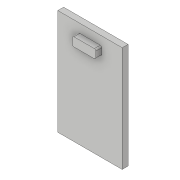
# Autodesk Inventor part: door
Saved by Autodesk Inventor 2017 (Build 210142000, 142)
## iProperties
Created: 2018-11-30
Part Number: door
Material: Generic
Document SubType Name: Modeling
Designer: jpb34
Density: 1 g/cm^3
Appearance: Default
Author: jpb34
Autodesk Inventor part; units mm, degrees
ref_plane "YZ Plane" through (0, 0, 0) normal (1, 0, 0) x (0, 1, 0)
ref_plane "XZ Plane" through (0, 0, 0) normal (0, 1, 0) x (-1, 0, 0)
ref_plane "XY Plane" through (0, 0, 0) normal (0, 0, 1) x (1, 0, 0)
sketch "Sketch1" plane through (0, 0, 0) normal (0, 0, 1) x (1, 0, 0)
  line L0 (-69.85, 114.3) -> (69.85, 114.3)
  line L1 (69.85, 114.3) -> (69.85, -114.3)
  line L2 (69.85, -114.3) -> (-69.85, -114.3)
  line L3 (-69.85, -114.3) -> (-69.85, 114.3)
  point P0 (0, 0)
  dimension "d0" = 139.7
  dimension "d1" = 228.6
  dimension "d2" = 114.3
  dimension "d3" = 69.85
  constraints: 8 end point, 2 parallel, 1 horizontal, 1 perpendicular
  measures "d0" distance of L0.start L0.end
  measures "d1" distance of L0.end L1.end
  measures "d2" distance from line of point (0, 0) L0
  measures "d3" distance from line of L1 point (0, 0)
extrude "Extrusion1" add sketch "Sketch1" along normal blind 12.7
sketch "Sketch2" plane through (0, 0, 12.7) normal (0, 0, 1) x (1, 0, 0)
  line L0 (-22.225, 95.25) -> (22.225, 95.25)
  line L1 (25.4, 92.075) -> (25.4, 79.375)
  line L2 (22.225, 76.2) -> (-22.225, 76.2)
  line L3 (-25.4, 79.375) -> (-25.4, 92.075)
  arc A0 (-22.225, 95.25) -> (-25.4, 92.075) centre (-22.225, 92.075) ccw
  arc A1 (-25.4, 79.375) -> (-22.225, 76.2) centre (-22.225, 79.375) ccw
  arc A2 (22.225, 76.2) -> (25.4, 79.375) centre (22.225, 79.375) ccw
  arc A3 (25.4, 92.075) -> (22.225, 95.25) centre (22.225, 92.075) ccw
  point P0 (0, 0)
  point P1 (25.4, 76.2)
  point P2 (25.4, 95.25)
  point P3 (-25.4, 76.2)
  dimension "d6" = 50.8
  dimension "d7" = 19.05
  dimension "d8" = 95.25
  dimension "d9" = 25.4
  dimension "d10" = 3.175
  constraints: 8 end point, 8 point on circle, 8 tangent, 6 point on line, 4 centre point, 3 equal radius, 2 parallel, 1 horizontal, 1 perpendicular
  measures "d6" distance of point (25.4, 76.2) point (-25.4, 76.2)
  measures "d7" distance of point (25.4, 95.25) point (25.4, 76.2)
  measures "d8" distance from line of point (0, 0) L0
  measures "d9" distance from line of point (0, 0) L1
  measures "d10" radius of A0
extrude "Extrusion2" add sketch "Sketch2" along normal blind 12.7
body "Solid1"
